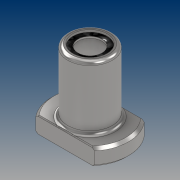
# Autodesk Inventor part: Dai_oc_truc_vit
Saved by Autodesk Inventor 2021 (Build 250183000, 183)
## iProperties
Created: 2024-04-08
Part Number: Dai_oc_truc_vit
Material: Stainless Steel, Austenitic
Document SubType Name: Modeling
Designer: Admin
Density: 8 g/cm^3
Appearance: Semi-Polished
Author: Admin
Autodesk Inventor part; units mm, degrees
ref_plane "YZ Plane" through (0, 0, 0) normal (1, 0, 0) x (0, 1, 0)
ref_plane "XZ Plane" through (0, 0, 0) normal (0, 1, 0) x (-1, 0, 0)
ref_plane "XY Plane" through (0, 0, 0) normal (0, 0, 1) x (1, 0, 0)
sketch "Sketch1" plane through (0, 0, 0) normal (0, 1, 0) x (-1, 0, 0)
  circle A0 centre (0, 0) radius 22.5
  line L0 (-17.2047, 14.5) -> (17.2047, 14.5)
  line L1 (17.2047, 14.5) -> (17.2047, -14.5)
  line L2 (17.2047, -14.5) -> (-17.2047, -14.5)
  line L3 (-17.2047, -14.5) -> (-17.2047, 14.5)
  line L4 (-17.2047, 14.5) -> (17.2047, -14.5) construction
  line L5 (17.2047, 14.5) -> (-17.2047, -14.5) construction
  circle A1 centre (0, 0) radius 10
  circle A2 centre (0, 0) radius 13
  dimension "d1" = 45
  dimension "d0" = 29
  dimension "d2" = 20
  dimension "d3" = 26
  constraints: 12 end point, 2 centre point, 2 coincident, 2 midpoint, 2 parallel, 1 horizontal, 1 perpendicular, 3 other
  measures "d0" distance between parallel lines of L0 L2
  measures "d2" diameter of A1
  measures "d3" diameter of A2
extrude "Extrusion1" add sketch "Sketch1" against normal blind 10 contours A0 L1 | L1 L2 L3 L0 | L3 A0 | A2
extrude "Extrusion2" add sketch "Sketch1" along normal blind 37 contours A2
fillet "Fillet1" radius 2 1 edges at (13, 0, 0)
ref_plane "Work Plane1" through (0, -7, 0) normal (0, -1, 0) x (1, 0, 0)
sketch "Sketch2" plane through (0, -7, 0) normal (0, -1, 0) x (1, 0, 0)
  circle A0 centre (0, 0) radius 10 projected
  circle A1 centre (0, 0) radius 7
  dimension "d10" = 14
  constraints: 1 centre point
  measures "d10" diameter of A1
extrude "Extrusion3" add sketch "Sketch2" along normal blind 1.25
ref_plane "Work Plane2" through (0, 35.75, 0) normal (0, 1, 0) x (1, 0, 0)
sketch "Sketch3" plane through (0, 35.75, 0) normal (0, 1, 0) x (1, 0, 0)
  circle A0 centre (0, 0) radius 13 projected
  circle A1 centre (0, 0) radius 10 projected
  circle A2 centre (0, 0) radius 7
  dimension "d14" = 14
  constraints: 1 centre point
  measures "d14" diameter of A2
extrude "Extrusion4" add sketch "Sketch3" against normal blind 1 contours A1
chamfer "Chamfer1" distance 0.5 angle 45 8 edges at (0, -10, 14.5) (0, -10, -14.5) (-10.5226, 0, 14.5) (0, 0.0635, 14.5) (10.5226, 0, 14.5) (-10.5226, 0, -14.5) (0, 0.0635, -14.5) (10.5226, 0, -14.5)
chamfer "Chamfer2" distance 1.5 angle 45 4 edges at (-22.5, -10, 0) (-22.5, 0, 0) (22.5, -10, 0) (22.5, 0, 0)
fillet "Fillet2" radius 2 1 edges at (13, 37, 0)
body "Solid1"
